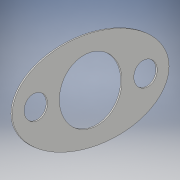
# Autodesk Inventor part: Component 29 (Flange Seal)
Saved by Autodesk Inventor 2018 (Build 220112000, 112)
## iProperties
Created: 2023-03-30
Part Number: Component 29 (Flange Seal)
Material: Generic
Document SubType Name: Modeling
Designer: Habib Mohamed
Density: 1 g/cm^3
Appearance: Default
Author: Habib Mohamed
Autodesk Inventor part; units mm, degrees
ref_plane "YZ Plane" through (0, 0, 0) normal (1, 0, 0) x (0, 1, 0)
ref_plane "XZ Plane" through (0, 0, 0) normal (0, 1, 0) x (-1, 0, 0)
ref_plane "XY Plane" through (0, 0, 0) normal (0, 0, 1) x (1, 0, 0)
sketch "Sketch1" plane through (0, 0, 0) normal (1, 0, 0) x (0, 1, 0)
  ellipse E0 centre (0, 0) end of major axis (0, -10) minor radius 6
  circle A0 centre (0, 7) radius 1.5
  circle A1 centre (0, -7) radius 1.5
  circle A2 centre (0, 0) radius 4
  line L0 (6, 0) -> (-6, 0) construction
  line L1 (0, 10) -> (0, -10) construction
  point P0 (0, 0)
  dimension "d0" = 3
  dimension "d1" = 8
  dimension "d3" = 7
  dimension "d4" = 7
  dimension "d5" = 20
  dimension "d6" = 12
  constraints: 4 end point, 3 centre point, 2 coincident, 2 midpoint, 2 vertical alignment, 1 equal radius, 1 horizontal, 1 vertical, 6 other
  measures "d0" diameter of A1
  measures "d1" diameter of A2
  measures "d3" distance of point (0, 0) A1.centre
  measures "d4" distance of A0.centre point (0, 0)
  measures "d5" distance of L1.start L1.end
  measures "d6" distance of L0.start L0.end
extrude "Extrusion1" add sketch "Sketch1" along normal blind 0.2
equation "\"d4\" = d3"
body "Solid1"
